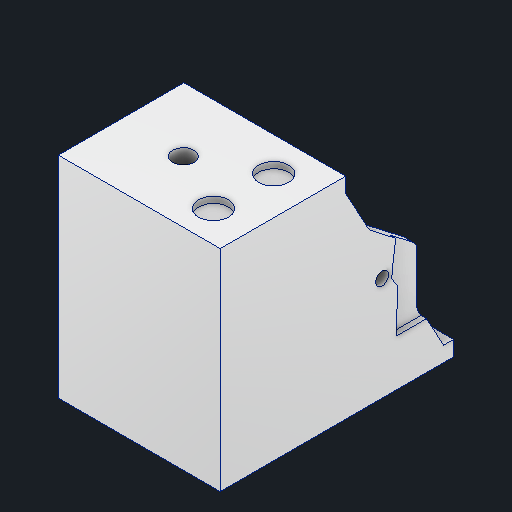
# Autodesk Inventor part: AC23[i3][L]
Saved by Autodesk Inventor 2024 (Build 280153000, 153)
## iProperties
Created: 2022-10-25
Part Number: AC23[i3][L]
Material: Aluminio 6061
Document SubType Name: Modeling
Designer: juanr
Density: 2.7 g/cm^3
Appearance: Aluminio - Plano
Author: juanr
Autodesk Inventor part; units mm, degrees
ref_plane "YZ Plane" through (0, 0, 0) normal (1, 0, 0) x (0, 1, 0)
ref_plane "XZ Plane" through (0, 0, 0) normal (0, 1, 0) x (-1, 0, 0)
ref_plane "XY Plane" through (0, 0, 0) normal (0, 0, 1) x (1, 0, 0)
sketch "Sketch1" plane through (0, 0, 0) normal (0, 1, 0) x (-1, 0, 0)
  line L0 (0, -25.5) -> (-34.15, -25.5)
  line L1 (-34.15, -25.5) -> (-34.15, 0)
  line L2 (-34.15, 0) -> (-34.15, 25.5)
  line L3 (-34.15, 25.5) -> (0, 25.5)
  line L4 (0, 25.5) -> (34.15, 25.5)
  line L5 (34.15, 25.5) -> (34.15, 0)
  line L6 (34.15, 0) -> (34.15, -25.5)
  line L7 (34.15, -25.5) -> (0, -25.5)
  point P0 (0, 0)
  constraints: 16 end point, 3 perpendicular, 2 point on line, 1 horizontal, 1 vertical
extrude "Extrusion1" add sketch "Sketch1" along normal blind 7
sketch "Sketch3" plane through (-34.15, 0, 25.5) normal (0, 0, 1) x (1, 0, 0)
  line L0 (0, 0) -> (0, -78.85)
  point P0 (34.15, 0)
  dimension "d7" = 78.85
  constraints: 2 end point, 1 vertical
  measures "d7" distance of L0.start L0.end
sketch "Sketch4" plane through (-34.15, 0, -25.5) normal (-1, 0, 0) x (0, 0, 1)
  line L0 (51, 0) -> (51, -78.85)
  line L1 (51, -78.85) -> (-39, -78.85)
  line L2 (-39, -78.85) -> (-39, -71.85)
  line L3 (0, 0) -> (-39, -71.85)
  line L4 (0, 0) -> (51, 0)
  point P0 (25.5, 0)
  dimension "d10" = 90
  dimension "d11" = 7
  constraints: 10 end point, 2 horizontal, 2 vertical
  measures "d10" distance of L0.end L1.end
  measures "d11" distance of L1.end L2.end
extrude "Extrusion2" add sketch "Sketch4" against normal blind 7
sketch "Sketch7" plane through (-27.15, 0, -25.5) normal (1, 0, 0) x (0, 0, -1)
  line L0 (-51, -78.85) -> (39, -78.85) projected
  line L1 (-51, -78.85) -> (39, -78.85)
  line L2 (39, -78.85) -> (39, -71.85) projected
  line L3 (39, -78.85) -> (39, -71.85)
  line L4 (39, -71.85) -> (-51, -71.85)
  line L5 (-51, 0) -> (-51, -78.85) projected
  line L6 (-51, -78.85) -> (-51, -71.85)
  point P0 (-25.5, 0)
  constraints: 8 end point, 2 perpendicular, 1 collinear, 1 horizontal, 1 point on line
sketch "Sketch8" plane through (0, 0, 0) normal (0, -1, 0) x (1, 0, 0)
  circle A0 centre (8.15, 0) radius 5 projected
  line L0 (8.15, 18.5) -> (34.15, 18.5)
  line L1 (34.15, 25.5) -> (34.15, -25.5) projected
  line L2 (8.15, 25.5) -> (34.15, 25.5)
  line L3 (8.15, 25.5) -> (-27.15, 25.5)
  line L4 (-27.15, 25.5) -> (-27.15, -25.5) projected
  line L5 (8.15, 18.5) -> (-27.15, 18.5)
  line L6 (34.15, 25.5) -> (34.15, 18.5)
  line L7 (-27.15, 25.5) -> (-27.15, 18.5)
  point P0 (0, 0)
  constraints: 12 end point, 2 collinear, 2 point on line, 1 horizontal, 1 parallel
extrude "Extrusion6" add sketch "Sketch7" along normal blind 58.5
extrude "Extrusion7" add sketch "Sketch8" along normal blind 78.75 contours L5 L4 L3 L2 L1 L0
sketch "Sketch9" plane through (31.35, 0, -25.5) normal (1, 0, 0) x (0, 0, -1)
  line L0 (-51, -78.75) -> (-51, 7) projected
  line L1 (-44, 0) -> (-44, -71.85) projected
  line L2 (-51, -78.75) -> (-44, -78.75)
  line L3 (-44, -78.75) -> (-44, -71.85)
  line L4 (-44, -71.85) -> (-51, -71.85)
  line L5 (-51, -71.85) -> (-51, -78.75)
  point P0 (-25.5, 0)
  constraints: 8 end point, 2 parallel, 1 horizontal, 1 perpendicular
extrude "Extrusion8" cut sketch "Sketch9" along normal blind 10
sketch "Sketch10" plane through (0, 7, 0) normal (0, 1, 0) x (1, 0, 0)
  point P0 (0, 0)
sketch "Boceto11" plane through (-34.15, -78.85, -64.5) normal (0, -1, 0) x (1, 0, 0)
  line L0 (0, 0) -> (65.5, 0) projected
  line L1 (65.5, 89.9985) -> (65.5, 0)
  line L2 (65.5, 0) -> (71.065, 0)
  line L3 (71.065, 0) -> (71.065, 89.9985)
  line L4 (71.065, 89.9985) -> (65.5, 89.9985)
  line L5 (65.5, 89.9985) -> (65.5, 95.8996)
  line L6 (65.5, 95.8996) -> (71.065, 89.9985)
  point P0 (34.15, 64.5)
  constraints: 12 end point, 3 perpendicular, 2 vertical
extrude "Extrusión9" cut sketch "Boceto11" against normal blind 100
sketch "Boceto12" plane through (31.35, 0, -25.5) normal (1, 0, 0) x (0, 0, -1)
  line L0 (-44, 0) -> (-44, -71.85) projected
  line L1 (-44, 0) -> (-44, -71.85)
  line L2 (39, -71.85) -> (39, -78.85) projected
  line L3 (-44, -71.85) -> (39, -71.85)
  line L4 (-44, 0) -> (0, 0) projected
  line L5 (39, -71.85) -> (0, 0)
  line L6 (0, 0) -> (-44, 0)
  point P0 (-25.5, 0)
  constraints: 8 end point, 1 collinear, 1 perpendicular, 1 vertical
extrude "Extrusión10" add sketch "Boceto12" against normal blind 7
sketch "Boceto13" plane through (-34.15, 7, -25.5) normal (-1, 0, 0) x (0, 0, 1)
  line L0 (0, -7) -> (0, 0) projected
  line L1 (44, -7) -> (0, -7) projected
  line L2 (0, -7) -> (44, -7)
  line L3 (44, -78.85) -> (-39, -78.85) projected
  line L4 (44, -7) -> (44, -78.85)
  line L5 (44, -78.85) -> (-39, -78.85)
  line L6 (-39, -78.85) -> (0, -7)
  point P0 (25.5, -7)
  constraints: 8 end point, 1 collinear, 1 horizontal, 1 perpendicular
extrude "Extrusión11" cut sketch "Boceto13" against normal blind 7
sketch "Boceto15" plane through (-34.15, 0, -25.5) normal (0, 0, -1) x (-1, 0, 0)
  point P0 (-34.15, 0)
sketch "Boceto19" plane through (-34.15, -78.85, -64.5) normal (0, -1, 0) x (1, 0, 0)
  line L0 (65.5, 90) -> (65.5, 0) projected
  line L1 (65.5, 0) -> (65.5, 40.9323)
  line L2 (81.7334, 40.9323) -> (65.5, 40.9323)
  line L3 (81.7334, 40.9323) -> (81.7334, 0)
  line L4 (81.7334, 0) -> (65.5, 0)
  point P0 (34.15, 64.5)
  constraints: 8 end point, 2 perpendicular, 1 point on line, 1 vertical
extrude "Extrusión17" cut sketch "Boceto19" against normal blind 100
sketch "Boceto20" plane through (24.35, 0, -25.5) normal (-1, 0, 0) x (0, 0, 1)
  line L0 (-29.1839, -53.7657) -> (-27.9516, -53.3206) projected
  line L1 (0, 0) -> (-39, -71.85) projected
  line L2 (-29.1839, -53.7657) -> (-27.8697, -51.3447)
  line L3 (-27.8697, -51.3447) -> (-27.9516, -53.3206) projected
  line L4 (-27.8697, -51.3447) -> (-27.9516, -53.3206)
  line L5 (-27.9516, -53.3206) -> (-29.1839, -53.7657)
  point P0 (25.5, 0)
  constraints: 6 end point, 2 collinear
extrude "Extrusión18" add sketch "Boceto20" against normal blind 7
sketch "Boceto21" plane through (24.35, 0, -25.5) normal (-1, 0, 0) x (0, 0, 1)
  point P0 (25.5, 0)
sketch "Boceto22" plane through (24.35, 0, -25.5) normal (-1, 0, 0) x (0, 0, 1)
  point P0 (25.5, 0)
sketch "Boceto24" plane through (31.35, 0, -25.5) normal (1, 0, 0) x (0, 0, -1)
  point P0 (-25.5, 0)
sketch "Boceto26" plane through (24.35, 0, -25.5) normal (-1, 0, 0) x (0, 0, 1)
  point P0 (25.5, 0)
sketch "Boceto27" plane through (31.35, 0, -25.5) normal (1, 0, 0) x (0, 0, -1)
  line L0 (-51, 7) -> (0, 7) projected
  line L1 (0, 7) -> (16.0227, 7)
  line L2 (16.0227, 7) -> (16.0227, -29.5187)
  line L3 (0, 0) -> (39, -71.85) projected
  line L4 (16.0227, -29.5187) -> (0, 0)
  line L5 (0, 0) -> (0, 7)
  point P0 (-25.5, 0)
  constraints: 8 end point, 1 horizontal, 1 parallel, 1 perpendicular, 1 point on line
extrude "Extrusión22" add sketch "Boceto27" against normal blind 7
sketch "Boceto28" plane through (24.35, 0, -25.5) normal (-1, 0, 0) x (0, 0, 1)
  line L0 (-16.0227, -29.5187) -> (-39, -71.85) projected
  line L1 (-16.0227, -29.5187) -> (0, 0)
  line L2 (0, 7) -> (-16.0227, 7) projected
  line L3 (0, 0) -> (0, 7)
  line L4 (0, 7) -> (-16.0227, 7)
  line L5 (-16.0227, 7) -> (-16.0227, -29.5187) projected
  line L6 (-16.0227, 7) -> (-16.0227, -29.5187)
  point P0 (25.5, 0)
  constraints: 8 end point, 3 perpendicular, 1 collinear
extrude "Extrusión23" cut sketch "Boceto28" against normal blind 7
sketch "Boceto29" plane through (31.35, 0, -25.5) normal (1, 0, 0) x (0, 0, -1)
  point P0 (-25.5, 0)
sketch "Boceto31" plane through (-34.15, -78.85, -64.5) normal (0, 0, -1) x (-1, 0, 0)
  line L0 (0, 7) -> (0, 0) projected
  line L1 (0, 0) -> (0, 1)
  line L2 (0, 1) -> (-65.5, 1)
  line L3 (-65.5, 0) -> (-65.5, 85.85) projected
  line L4 (-65.5, 1) -> (-64.5, 1)
  line L5 (-64.5, 1) -> (-64.5, 85.85)
  line L6 (0, 85.85) -> (-65.5, 85.85) projected
  line L7 (-64.5, 85.85) -> (0, 85.85)
  line L8 (0, 85.85) -> (0, 84.85)
  line L9 (0, 0) -> (0, 85.85) projected
  line L10 (0, 84.85) -> (-64.5, 84.85)
  line L11 (-64.5, 85.85) -> (-65.5, 85.85)
  line L12 (0, 0) -> (-65.5, 0) projected
  line L13 (-65.5, 85.85) -> (-65.5, 0)
  line L14 (-65.5, 0) -> (0, 0)
  point P0 (-34.15, 78.85)
  dimension "d84" = 1
  dimension "d85" = 1
  dimension "d86" = 1
  constraints: 20 end point, 6 point on line, 4 perpendicular, 1 horizontal, 1 parallel, 1 vertical
  measures "d84" distance of L0.end L1.end
  measures "d85" distance of L2.end L4.end
  measures "d86" distance of L7.end L8.end
extrude "Extrusión26" cut sketch "Boceto31" against normal blind 1000 contours L0 L12 L3 L2 | L10 L5 L6 L8 | L2 L3 L6 L5
sketch "Boceto32" plane through (-34.15, -71.85, 18.5) normal (-1, 0, 0) x (0, 0, 1)
  line L0 (-83, -6) -> (7, -6) projected
  line L1 (7, -6) -> (6, -6)
  line L2 (6, -6) -> (6, 77.85)
  line L3 (7, 77.85) -> (-44, 77.85) projected
  line L4 (7, -6) -> (7, 77.85) projected
  line L5 (6, 77.85) -> (7, 77.85)
  line L6 (7, 77.85) -> (7, -6)
  point P0 (-18.5, 71.85)
  dimension "d89" = 1
  constraints: 8 end point, 2 point on line, 1 collinear, 1 horizontal, 1 perpendicular
  measures "d89" distance of L0.end L1.end
extrude "Extrusión27" cut sketch "Boceto32" against normal blind 100
sketch "Boceto33" plane through (-34.15, 6, -25.5) normal (0, 1, 0) x (1, 0, 0)
  line L0 (0, 0) -> (0, -44) projected
  line L1 (0, 0) -> (0, -25.5)
  line L2 (0, -25.5) -> (25.3, -25.5)
  circle A0 centre (25.3, -25.5) radius 4.25
  point P0 (34.15, -25.5)
  dimension "d92" = 25.5
  dimension "d93" = 25.3
  dimension "d94" = 8.5
  constraints: 4 end point, 1 centre point, 1 coincident, 1 perpendicular, 1 point on line
  measures "d92" distance of L0.start L1.end
  measures "d93" distance of L1.end L2.end
  measures "d94" diameter of A0
extrude "Extrusión28" cut sketch "Boceto33" against normal blind 10
sketch "Boceto34" plane through (30.35, -77.85, -64.5) normal (1, 0, 0) x (0, 0, -1)
  point P0 (-64.5, 77.85)
sketch "Boceto35" plane through (30.35, -77.85, -64.5) normal (1, 0, 0) x (0, 0, -1)
  circle A0 centre (-24.4828, 41.285) radius 2.6
  point P0 (-64.5, 77.85)
  dimension "d101" = 5.2
  constraints: 1 centre point
  measures "d101" diameter of A0
extrude "Extrusión29" cut sketch "Boceto35" against normal blind 10
sketch "Boceto36" plane through (30.35, -77.85, -64.5) normal (1, 0, 0) x (0, 0, -1)
  point P0 (-64.5, 77.85)
sketch "Boceto37" plane through (30.35, -77.85, -64.5) normal (1, 0, 0) x (0, 0, -1)
  line L0 (-39, 77.85) -> (0, 6) projected
  line L1 (-12.3437, 28.741) -> (-12.3437, 48.1268)
  line L2 (-12.3437, 48.1268) -> (-28.4038, 58.3285)
  line L3 (-12.3437, 28.741) -> (-28.4038, 58.3285)
  point P0 (-64.5, 77.85)
  constraints: 6 end point, 2 point on line, 1 vertical
extrude "Extrusión30" add sketch "Boceto37" against normal blind 6
fillet "Empalme3" radius 10 3 edges at (27.35, -29.7232, -52.1563) (27.35, -49.109, -52.1563) (27.35, -19.5215, -36.0962)
sketch "Boceto38" plane through (30.35, -77.85, -64.5) normal (1, 0, 0) x (0, 0, -1)
  point P0 (-64.5, 77.85)
sketch "Boceto39" plane through (30.35, -77.85, -64.5) normal (1, 0, 0) x (0, 0, -1)
  line L0 (-6.8274, 18.5782) -> (-18.8698, 18.5782)
  line L1 (-18.8698, 18.5782) -> (-18.2969, 35.7502)
  line L2 (-18.2969, 35.7502) -> (-20.685, 39.2299)
  line L3 (-20.685, 39.2299) -> (-19.4909, 52.6668)
  line L4 (-26.2143, 56.9377) -> (-16.9818, 51.073) projected
  line L5 (-6.8274, 18.5782) -> (-5.5662, 48.0514)
  line L6 (-5.5662, 48.0514) -> (-19.4909, 52.6668)
  point P0 (-64.5, 77.85)
  constraints: 12 end point, 1 horizontal, 1 point on line
extrude "Extrusión31" cut sketch "Boceto39" against normal blind 2.2
fillet "Empalme4" radius 10 1 edges at (29.25, -25.1832, -45.0091)
sketch "Boceto40" plane through (24.35, 0, -25.5) normal (-1, 0, 0) x (0, 0, 1)
  line L0 (-26.6563, -35.218) -> (-26.6563, -46.57) projected
  line L1 (-26.6563, -35.218) -> (-24.0221, -30.4862) construction
  arc A0 (-12.7857, -20.9123) -> (-9.3588, -17.2419) centre (-18.1476, -12.4713) ccw projected
  line L2 (-24.0221, -30.4862) -> (-10.7107, -19.1566) construction
  spline S0 degree 2 poles (-26.6563, -35.218) (-24.0221, -30.4862) (-10.7107, -19.1566) knots 1 1 1 2 2 2
  line L3 (-26.6563, -35.218) -> (-10.7107, -35.218)
  line L4 (-10.7107, -35.218) -> (-10.7107, -19.1566)
  line L5 (-10.7107, -19.1566) -> (-26.6563, -19.1566)
  line L6 (-26.6563, -19.1566) -> (-26.6563, -35.218)
  point P0 (25.5, 0)
  point P1 (-10.7107, -19.1566)
  constraints: 8 end point, 2 parallel, 2 point on circle, 1 horizontal, 1 perpendicular, 3 other
extrude "Extrusión32" cut sketch "Boceto40" against normal blind 6 contours S0 L6 L5
fillet "Empalme5" radius 10 1 edges at (26.25, -35.218, -52.1563)
sketch "Boceto41" plane through (-34.15, -71.85, 18.5) normal (0, 1, 0) x (1, 0, 0)
  circle A0 centre (11.5, 71.5) radius 5 projected
  circle A1 centre (11.5, 71.5) radius 6
  line L0 (11.5, 71.5) -> (-12.5, 71.5)
  line L1 (-12.5, 71.5) -> (-12.5, 95.5)
  line L2 (-12.5, 95.5) -> (11.5, 95.5)
  line L3 (11.5, 95.5) -> (11.5, 71.5)
  line L4 (64.5, 76.1726) -> (64.5, 83) projected
  line L5 (64.5, 83) -> (64.5, 95.5)
  line L6 (64.5, 95.5) -> (11.5, 95.5)
  line L7 (0, 83) -> (0, -6) projected
  line L8 (0, -6) -> (-12.5, -6)
  line L9 (-12.5, -6) -> (-12.5, 71.5)
  line L10 (64.5, 83) -> (11.5, 83)
  line L11 (0, 83) -> (58.5, 83) projected
  point P0 (34.15, 18.5)
  dimension "d113" = 12
  dimension "d114" = 24
  dimension "d115" = 24
  constraints: 18 end point, 3 perpendicular, 2 horizontal, 2 parallel, 2 point on line, 1 centre point, 1 coincident, 1 vertical
  measures "d113" diameter of A1
  measures "d114" distance of L1.end L2.end
  measures "d115" distance of L0.end L1.end
extrude "Extrusión33" add sketch "Boceto41" against normal blind 6 contours L11 L7 L0 L1 L2 L3 | L3 L6 L5 L10 | L7 L8 L9 L0
sketch "Boceto43" plane through (30.35, 6, 24.5) normal (0, 1, 0) x (1, 0, 0)
  circle A0 centre (-39.2, 24.5) radius 4.25 projected
  line L0 (-39.2, 24.5) -> (-15.2, 24.5)
  line L1 (-15.2, 24.5) -> (-15.2, 12.5)
  line L2 (-15.2, 12.5) -> (-15.2, 36.5)
  circle A1 centre (-15.2, 36.5) radius 6
  circle A2 centre (-15.2, 12.5) radius 6
  point P0 (-30.35, 24.5)
  dimension "d123" = 24
  dimension "d124" = 12
  dimension "d125" = 24
  dimension "d126" = 12
  dimension "d127" = 12
  constraints: 6 end point, 2 centre point, 2 coincident, 1 horizontal, 1 perpendicular, 1 point on line
  measures "d123" distance of L0.start L0.end
  measures "d124" distance of L0.end L1.end
  measures "d125" distance of L1.end L2.end
  measures "d126" diameter of A1
  measures "d127" diameter of A2
extrude "Extrusión35" cut sketch "Boceto43" against normal blind 2.5 contours A1 | A2
sketch "Boceto44" plane through (24.35, 0, -25.5) normal (-1, 0, 0) x (0, 0, 1)
  line L0 (0, 0) -> (-9.3588, -17.2419) projected
  line L1 (-9.3588, -17.2419) -> (-30.5215, -33.5874)
  line L2 (-30.5215, -33.5874) -> (-30.5215, -56.2301)
  line L3 (-27.8675, -51.3405) -> (-39, -71.85) projected
  arc A0 (-12.666, -20.8351) -> (-9.3588, -17.2419) centre (-18.1476, -12.4713) ccw projected
  line L4 (-30.5215, -56.2301) -> (-9.3588, -17.2419)
  point P0 (25.5, 0)
  constraints: 6 end point, 1 point on line, 1 tangent, 1 vertical
extrude "Extrusión36" add sketch "Boceto44" against normal blind 6
sketch "Boceto45" plane through (30.35, 0, -25.5) normal (1, 0, 0) x (0, 0, -1)
  line L0 (18.315, -38.6201) -> (18.6875, -34.4282) projected
  line L1 (18.6875, -34.4282) -> (19.9402, -25.4146)
  line L2 (9.3588, -17.2419) -> (30.5215, -33.5874) projected
  line L3 (30.5215, -56.2301) -> (30.5215, -33.5874) projected
  line L4 (19.9402, -25.4146) -> (30.5215, -33.5874)
  line L5 (30.5215, -33.5874) -> (32.1519, -59.2336)
  line L6 (30.5215, -56.2301) -> (39, -71.85) projected
  line L7 (32.1726, -59.2718) -> (20.1302, -59.2718) projected
  line L8 (32.1726, -59.2718) -> (18.315, -38.6201)
  point P0 (-25.5, 0)
  constraints: 8 end point, 1 midpoint, 1 point on line
extrude "Extrusión37" cut sketch "Boceto45" against normal blind 2.2 contours L0 L1 L2 L3 L6 L8
fillet "Empalme7" radius 4 3 edges at (26.25, -33.5874, -56.0215) (27.35, -17.2419, -34.8588) (26.25, -56.2301, -56.0215)
sketch "Boceto46" plane through (-34.15, -71.85, 18.5) normal (0, 1, 0) x (1, 0, 0)
  line L0 (-12.5, -6) -> (0, -6) projected
  line L1 (0, -6) -> (0, 95.5)
  line L2 (-12.5, 95.5) -> (64.5, 95.5) projected
  line L3 (0, 95.5) -> (-12.5, 95.5)
  line L4 (-12.5, 95.5) -> (-12.5, -6)
  line L5 (-12.5, -6) -> (0, -6)
  point P0 (34.15, 18.5)
  constraints: 8 end point, 3 perpendicular, 1 vertical
extrude "Extrusión38" cut sketch "Boceto46" against normal blind 10
sketch "Boceto47" plane through (-34.15, -71.85, 18.5) normal (0, 1, 0) x (1, 0, 0)
  line L0 (0, 0) -> (0, -6) projected
  line L1 (0, 95.5) -> (26.5, 95.5)
  line L2 (26.5, 95.5) -> (26.5, 69)
  line L3 (26.5, 69) -> (0, 69)
  line L4 (0, 69) -> (0, 95.5)
  circle A0 centre (26.5, 69) radius 6
  point P0 (34.15, 18.5)
  dimension "d137" = 26.5
  dimension "d138" = 26.5
  dimension "d139" = 12
  constraints: 8 end point, 2 parallel, 1 centre point, 1 coincident, 1 horizontal, 1 perpendicular
  measures "d137" distance of L2.end L3.end
  measures "d138" distance of L1.end L2.end
  measures "d139" diameter of A0
extrude "Extrusión39" cut sketch "Boceto47" against normal blind 10 contours A0 L3 L2 | L2 L3 A0
sketch "Sketch48" plane through (-34.15, -71.85, 18.5) normal (0, 1, 0) x (1, 0, 0)
  circle A0 centre (26.5, 69) radius 6 projected
  line L0 (29.7126, 74.0675) -> (26.5, 69)
  circle A1 centre (26.5, 69) radius 18
  line L1 (8.5, 69) -> (8.5, 0)
  line L2 (0, 0) -> (58.5, 0) projected
  line L3 (0, 0) -> (8.5, 0)
  line L4 (26.5, 87) -> (64.5, 87)
  line L5 (64.5, 83) -> (64.5, 95.5) projected
  line L6 (0, 0) -> (0, 95.5) projected
  line L7 (64.5, 95.5) -> (0, 95.5)
  line L8 (0, 95.5) -> (0, 0)
  point P0 (34.15, 18.5)
  dimension "d142" = 36
  constraints: 12 end point, 2 point on circle, 2 point on line, 1 centre point, 1 coincident, 1 collinear, 1 parallel, 1 perpendicular, 1 vertical, 2 other
  measures "d142" diameter of A1
extrude "Extrusion40" cut sketch "Sketch48" against normal blind 10 contours A1 L1 L2 L6 L7 L5 L4
sketch "Sketch49" plane through (24.35, 0, 18.5) normal (0, 0, -1) x (-1, 0, 0)
  line L0 (58.5, -77.85) -> (50, -77.85) projected
  line L1 (58.5, -77.85) -> (50, -77.85)
  line L2 (50, -71.85) -> (0, -71.85) projected
  line L3 (50, -77.85) -> (50, -71.85)
  line L4 (50, -71.85) -> (58.5, -71.85)
  line L5 (58.5, -71.85) -> (58.5, -77.85)
  point P0 (24.35, 0)
  constraints: 8 end point, 3 perpendicular, 1 horizontal
extrude "Extrusion41" add sketch "Sketch49" along normal blind 20
fillet "Fillet8" radius 7 1 edges at (-34.15, -74.85, -1.5)
fillet "Fillet9" radius 2 1 edges at (-25.65, -74.85, -1.5)
sketch "Sketch50" plane through (28.15, -77.85, -64.5) normal (1, 0, 0) x (0, 0, -1)
  point P0 (-64.5, 77.85)
sketch "Sketch51" plane through (-34.15, -77.85, 24.5) normal (0, -1, 0) x (1, 0, 0)
  line L0 (64.5, -50) -> (64.5, 0) projected
  line L1 (64.5, 0) -> (-39.5, 0)
  line L2 (-39.5, 0) -> (-39.5, -120)
  line L3 (-39.5, -120) -> (64.5, -120)
  line L4 (64.5, -120) -> (64.5, 0)
  point P0 (34.15, -24.5)
  dimension "d149" = 104
  dimension "d150" = 120
  constraints: 8 end point, 2 parallel, 1 horizontal, 1 perpendicular
  measures "d149" distance of L3.end L2.end
  measures "d150" distance of L2.end L1.end
body "Solid1"
